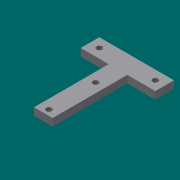
# Autodesk Inventor part: 知能ロボコンファン止め具
Saved by Autodesk Inventor 2013 (Build 170138000, 138)
## iProperties
Created: 2014-11-21
Part Number: 知能ロボコンファン止め具
Material: 一般
Document SubType Name: Modeling
Designer: horumo136
Density: 1 g/cm^3
Author: horumo136
Autodesk Inventor part; units mm, degrees
ref_plane "YZ Plane" through (0, 0, 0) normal (1, 0, 0) x (0, 1, 0)
ref_plane "XZ Plane" through (0, 0, 0) normal (0, 1, 0) x (-1, 0, 0)
ref_plane "XY Plane" through (0, 0, 0) normal (0, 0, 1) x (1, 0, 0)
sketch "スケッチ1" plane through (0, 0, 0) normal (0, 0, 1) x (1, 0, 0)
  line L0 (0, 0) -> (0, 10)
  line L1 (-20, 10) -> (20, 10)
  line L2 (20, 10) -> (20, 0)
  line L3 (20, 0) -> (-20, 0)
  line L4 (-20, 0) -> (-20, 10)
  line L5 (-20, 10) -> (20, 0) construction
  line L6 (20, 10) -> (-20, 0) construction
  line L7 (0, 5) -> (15, 5)
  line L8 (0, 5) -> (-15, 5)
  circle A0 centre (-15, 5) radius 1.5
  circle A1 centre (15, 5) radius 1.5
  line L9 (0, 0) -> (0, -12)
  line L10 (0, 0) -> (0, -37)
  circle A2 centre (0, -12) radius 1.5
  circle A3 centre (0, -37) radius 1.5
  line L11 (0, 0) -> (5, 0)
  line L12 (5, 0) -> (-5, 0)
  line L13 (-5, 0) -> (-5, -40)
  line L14 (-5, -40) -> (5, -40)
  line L15 (5, -40) -> (5, 0)
  dimension "d0" = 10
  dimension "d1" = 40
  dimension "d2" = 15
  dimension "d3" = 15
  dimension "d4" = 3
  dimension "d5" = 3
  dimension "d6" = 12
  dimension "d7" = 37
  dimension "d8" = 3
  dimension "d9" = 3
  dimension "d10" = 5
  dimension "d11" = 10
  dimension "d12" = 40
  constraints: 32 end point, 4 centre point, 4 coincident, 4 parallel, 4 perpendicular, 3 midpoint, 2 collinear, 2 horizontal, 1 point on line, 1 vertical
  measures "d0" distance of L0.start L0.end
  measures "d1" distance of L2.end L3.end
  measures "d2" distance of L7.start L7.end
  measures "d3" distance of L7.start L8.end
  measures "d4" diameter of A0
  measures "d5" diameter of A1
  measures "d6" distance of L0.start L9.end
  measures "d7" distance of L0.start L10.end
  measures "d8" diameter of A2
  measures "d9" diameter of A3
  measures "d10" distance of L0.start L11.end
  measures "d11" distance of L14.end L13.end
  measures "d12" distance of L13.end L12.end
extrude "押し出し1" add sketch "スケッチ1" along normal blind 4
